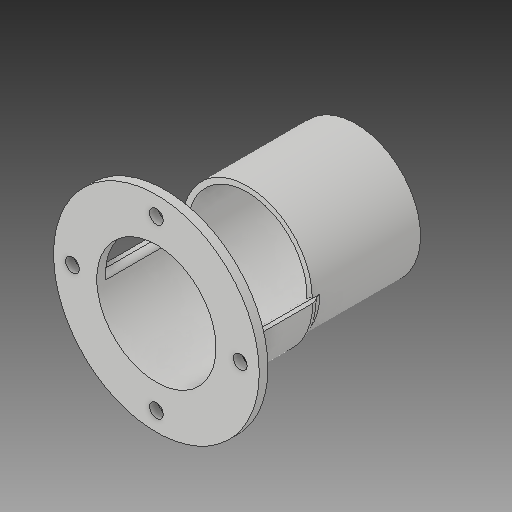
# Autodesk Inventor part: weapon motor inverted mount
Saved by Autodesk Inventor 2019 (Build 230136000, 136)
## iProperties
Created: 2017-12-10
Part Number: weapon motor inverted mount
Material: Generic
Document SubType Name: Modeling
Designer: rk_fe
Density: 1 g/cm^3
Appearance: Default
Author: rk_fe
Autodesk Inventor part; units mm, degrees
ref_plane "YZ Plane" through (0, 0, 0) normal (1, 0, 0) x (0, 1, 0)
ref_plane "XZ Plane" through (0, 0, 0) normal (0, 1, 0) x (-1, 0, 0)
ref_plane "XY Plane" through (0, 0, 0) normal (0, 0, 1) x (1, 0, 0)
sketch "Sketch1" plane through (0, 0, 0) normal (0, 0, 1) x (1, 0, 0)
  circle A0 centre (0, 0) radius 34.9504
  circle A1 centre (0, 0) radius 38.1
  dimension "d0" = 69.9008
  dimension "d1" = 76.2
  constraints: 2 centre point, 2 coincident
  measures "d0" diameter of A0
  measures "d1" diameter of A1
extrude "Extrusion2" add sketch "Sketch1" along normal blind 63.5
sketch "Sketch2" plane through (0, 0, 63.5) normal (0, 0, 1) x (1, 0, 0)
  circle A0 centre (0, 0) radius 34.9504 projected
  arc A1 (-34.9504, 0) -> (34.9504, 0) centre (0, 0) ccw
  circle A2 centre (0, 0) radius 38.1 projected
  arc A3 (-38.1, 0) -> (38.1, 0) centre (0, 0) ccw
  line L0 (-38.1, 0) -> (-34.9504, 0)
  line L1 (34.9504, 0) -> (38.1, 0)
  constraints: 8 point on circle, 4 end point, 2 centre point, 1 collinear, 1 horizontal
extrude "Extrusion3" add sketch "Sketch2" along normal blind 48.26 contours L1 A2 L0 A0 picked at (-20.6924, -30.48)
sketch "Sketch3" plane through (0, 0, 111.76) normal (0, 0, 1) x (1, 0, 0)
  circle A0 centre (0, 0) radius 34.9504
  circle A1 centre (0, 0) radius 60.325
  dimension "d9" = 69.9008
  dimension "d10" = 120.65
  constraints: 2 centre point, 2 coincident
  measures "d9" diameter of A0
  measures "d10" diameter of A1
extrude "Extrusion4" add sketch "Sketch3" along normal blind 5.08
sketch "Sketch4" plane through (0, 0, 111.76) normal (0, 0, -1) x (-1, 0, 0)
  circle A0 centre (0, 0) radius 38.1 projected
  line L0 (0, -38.1) -> (0, -60.325)
  circle A1 centre (0, 0) radius 60.325 projected
  line L1 (-38.1, 0) -> (-60.325, 0)
  line L2 (0, 38.1) -> (0, 60.325)
  line L3 (38.1, 0) -> (60.325, 0)
  circle A2 centre (0, -49.2125) radius 4.064
  circle A3 centre (-49.2125, 0) radius 4.064
  circle A4 centre (0, 49.2125) radius 4.064
  circle A5 centre (49.2125, 0) radius 4.064
  dimension "d13" = 8.128
  dimension "d14" = 8.128
  dimension "d15" = 8.128
  dimension "d16" = 8.128
  constraints: 8 end point, 8 point on circle, 4 centre point, 4 midpoint, 2 point on line, 1 horizontal, 1 perpendicular, 1 vertical
  measures "d13" diameter of A2
  measures "d14" diameter of A3
  measures "d15" diameter of A4
  measures "d16" diameter of A5
extrude "Extrusion5" cut sketch "Sketch4" against normal blind 12.7 contours A5 L3 | L3 A5 | A4 L2 | L2 A4 | A2 L0 | L0 A2 | A3 L1 | L1 A3
sketch "Sketch5" plane through (0, 0, 63.5) normal (0, 0, 1) x (1, 0, 0)
  line L0 (-34.9504, 0) -> (-38.1, 0) projected
  line L1 (-38.1, 0) -> (-40.64, 0)
  line L2 (38.1, 0) -> (34.9504, 0) projected
  line L3 (38.1, 0) -> (40.64, 0)
  arc A0 (-40.64, 0) -> (40.64, 0) centre (0, 0) ccw
  arc A1 (-38.1, 0) -> (38.1, 0) centre (0, 0) ccw projected
  dimension "d19" = 2.54
  dimension "d20" = 2.54
  constraints: 4 end point, 2 horizontal, 2 point on circle, 1 centre point
  measures "d19" distance of L0.end L1.end
  measures "d20" distance of L2.start L3.end
extrude "Extrusion6" add sketch "Sketch5" along normal blind 53.34
fillet "Fillet1" radius 5.08 1 edges at (0, -38.1, 63.5)
fillet "Fillet3" radius 5.08 1 edges at (0, -40.64, 63.5)
fillet "Fillet5" radius 3.175 2 edges at (-34.9504, 0, 87.63) (34.9504, 0, 87.63)
ref_plane "Work Plane1" through (0, 0, 34.417) normal (0, 0, -1) x (-1, 0, 0)
body "Solid2"
